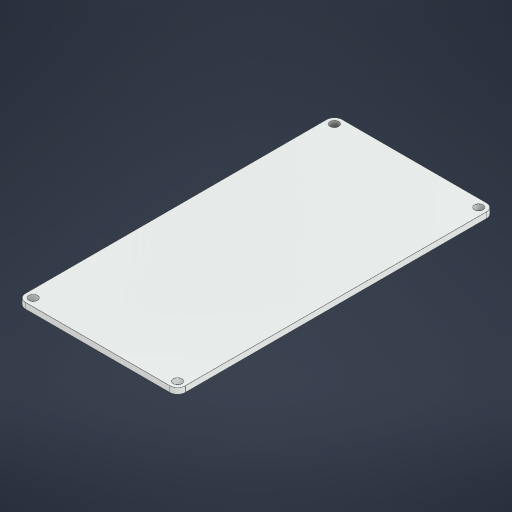
# Autodesk Inventor part: black_screen
Saved by Autodesk Inventor 2024.2 (Build 282272000, 272)
## iProperties
Created: 2025-05-21
Part Number: black_screen
Material: Generic
Document SubType Name: Modeling
Designer: Moe
Density: 1 g/cm^3
Appearance: Default
Author: Moe
Autodesk Inventor part; units mm, degrees
ref_plane "YZ Plane" through (0, 0, 0) normal (1, 0, 0) x (0, 1, 0)
ref_plane "XZ Plane" through (0, 0, 0) normal (0, 1, 0) x (-1, 0, 0)
ref_plane "XY Plane" through (0, 0, 0) normal (0, 0, 1) x (1, 0, 0)
sketch "Sketch1" plane through (0, 0, 0) normal (0, 1, 0) x (-1, 0, 0)
  line L0 (2, 0) -> (39.392, 0)
  line L1 (41.392, -2) -> (41.392, -80)
  line L2 (39.392, -82) -> (2, -82)
  line L3 (0, -80) -> (0, -2)
  arc A0 (41.392, -2) -> (39.392, 0) centre (39.392, -2) ccw
  arc A1 (39.392, -82) -> (41.392, -80) centre (39.392, -80) ccw
  arc A2 (0, -80) -> (2, -82) centre (2, -80) ccw
  arc A3 (2, 0) -> (0, -2) centre (2, -2) ccw
  circle A4 centre (39.386, -2.006) radius 1.1
  circle A5 centre (39.386, -79.994) radius 1.1
  circle A6 centre (2.006, -2.006) radius 1.1
  circle A7 centre (2.006, -79.994) radius 1.1
  point P0 (0, 0)
  point P1 (41.392, -82)
  point P2 (41.392, 0)
  point P3 (0, -82)
  dimension "d0" = 41.392
  dimension "d1" = 82
  dimension "d2" = 2
  dimension "d3" = 2.2
  dimension "d5" = 2.006
  dimension "d6" = 2.006
  dimension "d7" = 2.2
  dimension "d8" = 2.006
  dimension "d9" = 2.006
  dimension "d10" = 2.2
  dimension "d11" = 2.006
  dimension "d12" = 2.006
  dimension "d13" = 2.2
  dimension "d14" = 2.006
  dimension "d15" = 2.006
  dimension "d16" = 37.386
  constraints: 8 centre point, 8 end point, 8 point on circle, 8 point on line, 8 tangent, 3 equal radius, 2 parallel, 1 horizontal, 1 perpendicular
  measures "d0" distance of point (41.392, -82) point (0, -82)
  measures "d1" distance of point (41.392, 0) point (41.392, -82)
  measures "d2" radius of A0
  measures "d3" diameter of A4
  measures "d5" distance from line of L1 A4.centre
  measures "d6" distance from line of L0 A4.centre
  measures "d7" diameter of A5
  measures "d8" distance from line of L1 A5.centre
  measures "d9" distance from line of L2 A5.centre
  measures "d10" diameter of A6
  measures "d11" distance from line of L3 A6.centre
  measures "d12" distance from line of L0 A6.centre
  measures "d13" diameter of A7
  measures "d14" distance from line of L3 A7.centre
  measures "d15" distance from line of L2 A7.centre
  measures "d16" distance of A3.centre A4.centre
extrude "Extrusion1" add sketch "Sketch1" along normal blind 1.5
body "Solid1"
